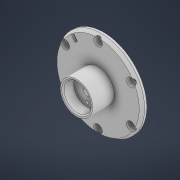
# Autodesk Inventor part: Ring Cover
Saved by Autodesk Inventor 2021 (Build 250183000, 183)
## iProperties
Created: 2025-03-19
Part Number: Ring Cover
Material: Generic
Document SubType Name: Modeling
Designer: rocke
Density: 0.538702 g/cm^3
Appearance: Default
Mass: 23.61 g
Surface Area: 169.275 cm^2
Volume: 43.8275 cm^3
Author: rocke
Autodesk Inventor part; units mm, degrees
ref_plane "YZ Plane" through (0, 0, 0) normal (1, 0, 0) x (0, 1, 0)
ref_plane "XZ Plane" through (0, 0, 0) normal (0, 1, 0) x (-1, 0, 0)
ref_plane "XY Plane" through (0, 0, 0) normal (0, 0, 1) x (1, 0, 0)
sketch "Sketch1" plane through (0, 0, 0) normal (0, 0, 1) x (1, 0, 0)
  circle A0 centre (0, 0) radius 40
  dimension "d0" = 80
  constraints: 1 centre point, 1 coincident
  measures "d0" diameter of A0
extrude "Extrusion1" add sketch "Sketch1" along normal blind 5
sketch "Sketch2" plane through (0, 0, 5) normal (0, 0, 1) x (1, 0, 0)
  point P0 (0, 0)
  point P1 (0, 35)
  dimension "d3" = 35
  measures "d3" distance of point (0, 0) point (0, 35)
hole "Hole1" at (0, 35, 5) direction (0, 0, -1) diameter 4.3 end through all counterbore diameter 8 counterbore depth 3.5 clearance for "Socket Head Cap Screw" size "M4" standard "Ansi Metric M Profile"
pattern_circular "Circular Pattern1" count 6 over 360 about axis through (0, 0, 0) along (0, 0, 1) of "Hole1"
chamfer "Chamfer1" distance 2 distance2 3 1 edges at (-40, 0, 5) measured on face at (-39.5, 0, 5)
sketch "Sketch3" plane through (0, 0, 5) normal (0, 0, -1) x (-1, 0, 0)
  circle A0 centre (0, 0) radius 30
  dimension "d17" = 60
  constraints: 1 centre point, 1 coincident
  measures "d17" diameter of A0
sketch "Sketch6" plane through (0, 0, 0) normal (0, 0, -1) x (-1, 0, 0)
  point P0 (0, 0)
sketch "Sketch7" plane through (0, 0, 5) normal (0, 0, 1) x (1, 0, 0)
  circle A0 centre (0, 0) radius 3.575 projected
  circle A1 centre (0, 0) radius 12.6
  circle A2 centre (0, 0) radius 15
  dimension "d32" = 25.2
  dimension "d33" = 30
  constraints: 2 centre point, 2 coincident
  measures "d32" diameter of A1
  measures "d33" diameter of A2
extrude "Extrusion5" add sketch "Sketch7" along normal blind 20 contours A0 | A1 | A2
sketch "Sketch10" plane through (0, 0, 0) normal (0, 0, -1) x (-1, 0, 0)
  circle A0 centre (0, 0) radius 15 projected
  circle A1 centre (0, 0) radius 30
  dimension "d44" = 60
  constraints: 1 centre point, 1 coincident
  measures "d44" diameter of A1
extrude "Extrusion7" cut sketch "Sketch10" against normal blind 2 contours A0 | A1
sketch "Sketch11" plane through (0, 0, 2) normal (0, 0, -1) x (-1, 0, 0)
  circle A0 centre (0, 0) radius 12.75
  dimension "d47" = 25.5
  constraints: 1 centre point, 1 coincident
  measures "d47" diameter of A0
extrude "Extrusion8" cut sketch "Sketch11" against normal blind 8.5
sketch "Sketch5" plane through (0, 0, 10.5) normal (0, 0, -1) x (-1, 0, 0)
  point P0 (0, 0)
  point P1 (0, 8.5)
  point P2 (0, -8.5)
  dimension "d23" = 8.5
  dimension "d24" = 8.5
  measures "d23" distance of point (0, 8.5) point (0, 0)
  measures "d24" distance of point (0, 0) point (0, -8.5)
hole "Hole2" at (0, 8.5, 10.5) at (0, -8.5, 10.5) direction (0, 0, 1) diameter 3.2 end through all counterbore diameter 6.5 counterbore depth 3 clearance for "Socket Head Cap Screw" size "M3" standard "Ansi Metric M Profile"
sketch "Sketch12" plane through (0, 0, 10.5) normal (0, 0, -1) x (-1, 0, 0)
  circle A0 centre (0, 0) radius 3.575
  dimension "d50" = 7.15
  constraints: 1 centre point, 1 coincident
  measures "d50" diameter of A0
extrude "Extrusion9" cut sketch "Sketch12" against normal through all
sketch "Sketch13" plane through (0, 0, 25) normal (0, 0, 1) x (1, 0, 0)
  circle A0 centre (0, 0) radius 3.575 projected
  circle A1 centre (0, 0) radius 12.575
  dimension "d53" = 25.15
  constraints: 1 centre point, 1 coincident
  measures "d53" diameter of A1
extrude "Extrusion10" cut sketch "Sketch13" against normal blind 10 contours A0 | A1
chamfer "Chamfer2" distance 1 angle 45 1 edges at (-12.575, 0, 25)
chamfer "Chamfer3" distance 1 angle 45 1 edges at (12.75, 0, 2)
sketch "Sketch14" plane through (0, 0, 0) normal (0, 0, -1) x (-1, 0, 0)
  arc A0 (31.3167, 20.9212) -> (1.7537, 37.6212) centre (0, 0) ccw
  line L0 (0, 0) -> (40, 0) construction
  line L1 (21.4926, 23.7527) -> (24.6091, 28.2845)
  line L2 (24.6091, 28.2845) -> (17.6054, 33.101)
  line L3 (17.6054, 33.101) -> (14.4889, 28.5691)
  line L4 (14.4889, 28.5691) -> (21.4926, 23.7527)
  line L5 (21.4926, 23.7527) -> (17.6054, 33.101) construction
  line L6 (24.6091, 28.2845) -> (14.4889, 28.5691) construction
  line L7 (17.002, 26.8409) -> (20.1185, 31.3727)
  line L8 (22.1372, 29.9845) -> (19.0207, 25.4526)
  line L9 (14.8714, 29.1253) -> (17.223, 32.5448)
  line L10 (17.223, 32.5448) -> (19.736, 30.8165)
  line L11 (19.736, 30.8165) -> (17.3845, 27.3971)
  line L12 (17.3845, 27.3971) -> (14.8714, 29.1253)
  line L13 (19.549, 28.4268) -> (16.0472, 30.8351)
  line L14 (17.3845, 27.3971) -> (17.223, 32.5448)
  line L15 (14.8714, 29.1253) -> (19.736, 30.8165)
  line L16 (0, 0) -> (17.3037, 29.9709)
  line L17 (0, 0) -> (19.549, 28.4268)
  point P0 (19.736, 30.8165)
  point P1 (17.3845, 27.3971)
  dimension "d62" = 8.5
  dimension "d63" = 5.5
  dimension "d64" = 34.5
  dimension "d65" = 3.05
  dimension "d66" = 3
  dimension "d67" = 4.15
  dimension "d68" = 60
  constraints: 36 end point, 6 point on line, 5 parallel, 5 perpendicular, 4 midpoint, 2 point on circle, 1 centre point, 1 coincident, 1 collinear, 1 horizontal, 1 other
  measures "d62" distance between parallel lines of L1 L3
  measures "d63" distance between parallel lines of L4 L2
  measures "d64" distance of L0.start L13.start
  measures "d65" distance between parallel lines of L3 L7
  measures "d66" distance between parallel lines of L1 L8
  measures "d67" distance between parallel lines of L12 L10
  measures "d68" angle of L0 L16
extrude "Extrusion11" cut sketch "Sketch14" against normal through all contours L4 L8 L2 L1
sketch "Sketch15" plane through (0, 0, 0) normal (1, 0, 0) x (0, 1, 0)
  line L0 (0, 0) -> (0, 25)
  line L1 (15, 25) -> (-15, 25) projected
  line L2 (-16.5641, 5) -> (16.5641, 5) projected
  circle A0 centre (0, 6.5) radius 1.4
  dimension "d71" = 1.5
  dimension "d72" = 2.8
  constraints: 2 end point, 1 centre point, 1 coincident, 1 midpoint, 1 point on line
  measures "d71" distance from line of L2 point (0, 6.5)
  measures "d72" diameter of A0
extrude "Extrusion12" cut sketch "Sketch15" against normal through all
equation "\"d32\" = MOTOR_OD + TRANSITION"
equation "\"d44\" = RING_OD - 2 * RING_WALL_THICKNESS"
equation "\"d53\" = MOTOR_OD + iNTERFERENCE"
equation "\"MOTOR_OD\" = 25"
equation "\"CLEARANCE\" = 0.3"
equation "\"TRANSITION\" = 0.2"
equation "\"iNTERFERENCE\" = 0.15"
equation "\"RING_OD\" = 80"
equation "\"RING_WALL_THICKNESS\" = 10"
body "Solid1"
